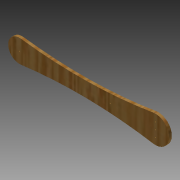
# Autodesk Inventor part: segment1b
Saved by Autodesk Inventor 2013 (Build 170138000, 138)
## iProperties
Created: 2014-10-09
Part Number: segment1b
Material: Generic
Document SubType Name: Modeling
Designer: Masta
Density: 1 g/cm^3
Author: Masta
Autodesk Inventor part; units mm, degrees
ref_plane "YZ Plane" through (0, 0, 0) normal (1, 0, 0) x (0, 1, 0)
ref_plane "XZ Plane" through (0, 0, 0) normal (0, 1, 0) x (-1, 0, 0)
ref_plane "XY Plane" through (0, 0, 0) normal (0, 0, 1) x (1, 0, 0)
sketch "Sketch1" plane through (0, 0, 0) normal (0, 1, 0) x (-1, 0, 0)
  line L0 (0, 0) -> (100, 0) construction
  line L1 (0, 0) -> (0, 15) construction
  line L2 (0, 0) -> (0, -15) construction
  arc A0 (4.8677, 29.6025) -> (4.8677, -29.6025) centre (0, 0) ccw
  line L3 (100, 0) -> (300, 0) construction
  arc A1 (4.8677, 29.6025) -> (296.7591, 24.789) centre (167.125, 1016.3509) ccw
  arc A2 (296.7591, -24.789) -> (4.8677, -29.6025) centre (167.125, -1016.3509) ccw
  arc A3 (296.7591, -24.789) -> (296.7591, 24.789) centre (300, 0) ccw
  dimension "d0" = 100
  dimension "d1" = 15
  dimension "d2" = 60
  dimension "d3" = 300
  dimension "d10" = 1000
  dimension "d11" = 25
  constraints: 8 end point, 8 point on circle, 7 coincident, 4 centre point, 3 symmetric about line, 2 collinear, 2 perpendicular, 2 tangent, 1 horizontal, 1 other
  measures "d0" distance of L0.start L0.end
  measures "d1" distance of L1.start L1.end
  measures "d2" diameter of A0
  measures "d3" distance of L1.start L3.end
  measures "d10" radius of A1
  measures "d11" radius of A3
extrude "Extrusion1" add sketch "Sketch1" along normal blind 6
hole "Hole1" at (0, 0, 0) at (-100, 0, 0) at (0, 0, 15) at (0, 0, -15) at (-300, 0, 0) direction (0, 1, 0) diameter 3 end through all
body "Solid1"
